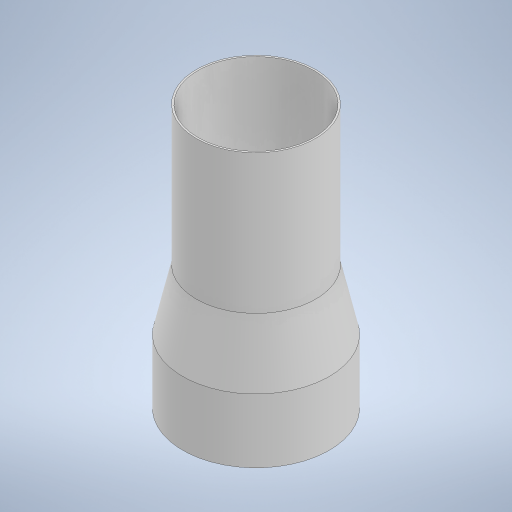
# Autodesk Inventor part: BottomTubeUp
Saved by Autodesk Inventor 2023.2 (Build 272271030, 271C)
## iProperties
Created: 2023-02-12
Part Number: BottomTubeUp
Material: Generic
Document SubType Name: Modeling
Designer: Lukas
Density: 1 g/cm^3
Appearance: Default
polomer: 33.200 mm
drazka: 50.000 mm
pcb: 66.000 mm
tvc_vyska: 16.000 mm
vyska_motor: 39.000 mm
tloustka: 2.000 mm
vyska: 200.000 mm
Author: Lukas
Autodesk Inventor part; units mm, degrees
ref_plane "YZ Plane" through (0, 0, 0) normal (1, 0, 0) x (0, 1, 0)
ref_plane "XZ Plane" through (0, 0, 0) normal (0, 1, 0) x (-1, 0, 0)
ref_plane "XY Plane" through (0, 0, 0) normal (0, 0, 1) x (1, 0, 0)
sketch "Sketch1" plane through (0, 0, 0) normal (1, 0, 0) x (0, 1, 0)
  line L0 (56.0515, -34.3) -> (106.0515, -34.3)
  line L1 (106.0515, -34.3) -> (106.0515, -35.3)
  line L2 (-80.6517, 0) -> (137.1687, 0) projected
  line L3 (25.6363, -32.7369) -> (-12.0345, -41.2096)
  line L4 (-11.7588, -43.3) -> (23.8103, -35.3)
  line L5 (23.8103, -35.3) -> (106.0515, -35.3)
  line L6 (-11.7588, -43.3) -> (-46.9485, -43.3)
  line L7 (56.0515, -34.3) -> (56.0515, -33.2)
  line L8 (56.0515, -33.2) -> (25.6363, -33.2)
  line L9 (25.6363, -33.2) -> (25.6363, -32.7369)
  line L10 (-12.0345, -41.2096) -> (-12.0345, -42.3)
  line L11 (-12.0345, -42.3) -> (-48.5345, -42.3)
  line L12 (-48.5345, -42.3) -> (-49.5345, -42.3)
  line L13 (-49.5345, -42.3) -> (-49.5345, -43.3)
  line L14 (-49.5345, -43.3) -> (-46.9485, -43.3)
  point P0 (0, 0)
  point P1 (106.0515, -34.8)
  dimension "d49" = 2.1
  dimension "d51" = 34.3
  dimension "d70" = 2.1
  dimension "d71" = 50
  dimension "d73" = 1
  dimension "d74" = 42.3
  dimension "d75" = 1
  dimension "d76" = 37.5
  dimension "d77" = 1
  dimension "d78" = 33.2
  constraints: 28 end point, 4 perpendicular, 2 collinear, 2 horizontal, 2 vertical, 1 midpoint, 1 parallel
  measures "d49" distance between parallel lines of L4 L3
  measures "d51" distance between parallel lines of L2 L0
  measures "d70" distance between parallel lines of L5 L8
  measures "d71" distance between parallel lines of L1 L7
  measures "d73" distance between parallel lines of L5 L0
  measures "d74" distance between parallel lines of L2 L11
  measures "d75" distance of L12.end L11.end
  measures "d76" distance between parallel lines of L10 L13
  measures "d77" distance between parallel lines of L6 L11
  measures "d78" distance between parallel lines of L2 L8
revolve "Revolution1" add sketch "Sketch1" angle 360 about axis through (0, -10, 0) along (0, 1, 0)
equation "\"gap\" = 0.1"
body "Solid1"
